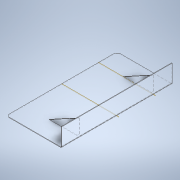
# Autodesk Inventor part: 21015-22-1-6- Work Shelves
Saved by Autodesk Inventor 2022 (Build 260153000, 153)
## iProperties
Created: 2021-06-17
Part Number: 21015-22-1-6- Work Shelves
Material: Steel, Carbon
Document SubType Name: Sheet Metal
Designer: Skynet
Density: 7.85 g/cm^3
Sheet Metal Rule: Default
Appearance: Semi-Polished
Author: Skynet
Autodesk Inventor part; units mm, degrees
ref_plane "YZ Plane" through (0, 0, 0) normal (1, 0, 0) x (0, 1, 0)
ref_plane "XZ Plane" through (0, 0, 0) normal (0, 1, 0) x (-1, 0, 0)
ref_plane "XY Plane" through (0, 0, 0) normal (0, 0, 1) x (1, 0, 0)
sketch "Sketch1" plane through (0, 0, 0) normal (0, 1, 0) x (-1, 0, 0)
  line L0 (0, 0) -> (304.8, 0)
  line L1 (304.8, 0) -> (304.8, -609.6)
  line L2 (304.8, -609.6) -> (0, -609.6)
  line L3 (0, -609.6) -> (0, 0)
  dimension "d0" = 609.6
  dimension "d1" = 304.8
  measures "d0" distance of L0.end L1.end
  measures "d1" distance of L0.start L0.end
extrude "Plate1" add sketch "Sketch1" along normal blind 3.175
sketch "Sketch2" plane through (-3.175, 0, -609.6) normal (1, 0, 0) x (0, 1, 0)
  line L0 (0, 609.6) -> (0, 0)
  line L1 (0, 0) -> (101.6, 0)
  line L2 (101.6, 0) -> (101.6, 609.6)
  line L3 (101.6, 609.6) -> (0, 609.6)
  constraints: 6 end point, 1 horizontal, 1 perpendicular, 1 vertical
edge flange "Flange1" height 101.6 angle 90 thickness 3.175 bend radius 3.175 thickness toward (1, 0, 0) relief tear relief width 3.175 relief depth 1.5875 edges at (0, 3.175, -304.8) wall of the first edge with corners at (-3.175, 0, 0) (-3.175, 0, -609.6) (-3.175, 101.6, -609.6) (-3.175, 101.6, 0)
bend "Bend1"
corner "Corner1"
chamfer "Chamfer1" distance 12.7 angle 45 2 edges at (-304.8, 1.5875, -609.6) (-304.8, 1.5875, 0)
ref_plane "Work Plane1" through (-6.35, 0, -508) normal (0, 0, -1) x (-1, 0, 0)
sketch "Sketch3" plane through (-6.35, 0, -508) normal (0, 0, -1) x (-1, 0, 0)
  line L0 (-3.175, 6.35) -> (-3.175, 101.6)
  line L1 (-3.175, 15.875) -> (9.525, 3.175)
  line L2 (285.75, 3.175) -> (0, 3.175)
  line L3 (161.925, 3.175) -> (-3.175, 92.075)
  line L4 (-3.175, 92.075) -> (-3.175, 15.875)
  line L5 (9.525, 3.175) -> (161.925, 3.175)
  point P0 (-6.35, 0)
  dimension "d17" = 152.4
  dimension "d18" = 76.2
  dimension "d19" = 12.7
  dimension "d20" = 135
  measures "d17" distance of L3.start L1.end
  measures "d18" distance of L1.start L3.end
  measures "d19" distance from line of L0 L1.end
  measures "d20" angle of L2 L1
sheet face with bend "Face2" sketch "Sketch3" thickness 3.175 toward (0, 0, -1) bend radius 3.175
bend "Bend2"
ref_plane "Work Plane2" through (-6.35, 0, -304.8) normal (0, 0, -1) x (-1, 0, 0)
mirror "Mirror1" about plane through (-6.35, 0, -304.8) normal (0, 0, -1)
equation "\"d2\" = Thickness"
equation "\"d3\" = BendReliefWidth"
equation "\"d4\" = BendReliefDepth"
equation "\"d5\" = MinimumRemnant"
equation "\"d6\" = TransitionRadius"
equation "\"d9\" = BendRadius"
equation "\"d10\" = CornerReliefSize"
equation "\"d11\" = GapSize"
equation "\"d12\" = JacobiRadiusSize"
equation "\"d21\" = BendRadius"
equation "\"d22\" = BendReliefWidth"
equation "\"d24\" = MinimumRemnant"
equation "\"d23\" = BendReliefDepth"
equation "\"d25\" = TransitionRadius"
equation "\"BendRadius\" = Thickness"
equation "\"BendReliefWidth\" = Thickness"
equation "\"BendReliefDepth\" = 0.5 * Thickness"
equation "\"CornerReliefSize\" = 4 * Thickness"
equation "\"MinimumRemnant\" = 2 * Thickness"
equation "\"TransitionRadius\" = BendRadius"
equation "\"JacobiRadiusSize\" = BendRadius"
equation "\"GapSize\" = Thickness"
equation "\"Thickness\" = 3.175"
body "Solid1"
